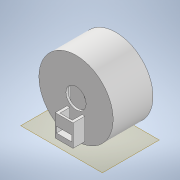
# Autodesk Inventor part: Crank
Saved by Autodesk Inventor 2022.2 (Build 262287000, 287)
## iProperties
Created: 2022-08-12
Part Number: Crank
Material: Generic
Document SubType Name: Modeling
Designer: Ilewicz
Density: 1 g/cm^3
Appearance: Default
r_crank: 15,000 mm
h_tool_holder: 4,000 mm
h_screw_plate: 0,800 mm
r_tool: 2,500 mm
Author: Ilewicz
Autodesk Inventor part; units mm, degrees
ref_plane "YZ Plane" through (0, 0, 0) normal (1, 0, 0) x (0, 1, 0)
ref_plane "XZ Plane" through (0, 0, 0) normal (0, 1, 0) x (-1, 0, 0)
ref_plane "XY Plane" through (0, 0, 0) normal (0, 0, 1) x (1, 0, 0)
derived "Motor.ipt"
sketch "Sketch1" plane through (0, 0, 0) normal (0, 0, 1) x (1, 0, 0)
  line L0 (-3.1964, 3.5) -> (-3.1964, -5.5) construction
  arc A0 (-1.1964, 3.4987) -> (-3.1964, 1.5) centre (-3.1964, 3.5) ccw construction
  line L1 (-5.6964, -1) -> (-5.6964, -3) construction
  line L2 (-0.6964, -3) -> (-0.6964, -1) construction
  arc A1 (-0.6964, -1) -> (-5.6964, -1) centre (-3.1964, -1) ccw construction
  circle A2 centre (-3.1964, 3.5) radius 1.1
  line L3 (2.1036, -3) -> (2.1036, 0)
  arc A3 (4.3036, 0) -> (2.1036, 0) centre (3.2036, 0) ccw
  line L4 (4.3036, 0) -> (4.3036, -3)
  arc A4 (2.1036, -3) -> (4.3036, -3) centre (3.2036, -3) ccw
  line L5 (0.1508, 2.1505) -> (5.7036, 2.1505)
  arc A5 (-1.1964, 3.4987) -> (0.1508, 2.1505) centre (0.1508, 3.4977) ccw
  arc A6 (-1.1964, 3.4987) -> (-3.1964, 1.5) centre (-3.1964, 3.5) ccw
  arc A7 (0.7036, -0.5) -> (-1.2964, 1.5) centre (-1.2964, -0.5) ccw
  line L6 (0.7036, -0.5) -> (0.7036, -3)
  arc A8 (0.7036, -3) -> (5.7036, -3) centre (3.2036, -3) ccw
  line L7 (5.7036, -3) -> (5.7036, 2.1505)
  circle A9 centre (-3.1964, 3.5) radius 1.6 construction
  spline S0 degree 3 poles (-0.0964, 1.1) (-0.2709, 1.2308) (-0.4689, 1.3337) (-0.8824, 1.4687) (-1.0974, 1.5) (-1.2964, 1.5) knots 0 0 0 0 0.5 0.5 1 1 1 1
  line L8 (-3.1964, 1.5) -> (-1.2964, 1.5)
  line L9 (0.4036, -1) -> (0.4036, -11.0616)
  line L10 (-6.7964, -11.0616) -> (-6.7964, -1)
  line L11 (-6.7964, -1) -> (0.4036, -1)
  arc A10 (-6.7964, -11.0616) -> (0.4036, -11.0616) centre (-3.1964, 3.5) ccw
  line L12 (-3.1964, -12.8219) -> (-3.1964, 17.006)
  line L13 (-0.6964, -3) -> (-5.6964, -3) construction
  line L14 (-5.6964, -3) -> (-0.6964, -3) construction
  line L15 (-0.6964, -3) -> (-0.6964, -5.5) construction
  line L16 (-0.6964, -5.5) -> (-5.6964, -5.5) construction
  line L17 (-5.6964, -5.5) -> (-5.6964, -3) construction
  line L18 (-6.2964, -7.9) -> (-0.0964, -7.9)
  line L19 (-0.0964, -7.9) -> (-0.0964, -5.5)
  line L20 (-0.0964, -5.5) -> (-6.2964, -5.5)
  line L21 (-6.2964, -5.5) -> (-6.2964, -7.9)
  line L22 (-6.7964, -9.9) -> (0.4036, -9.9)
  point P0 (0, 0)
  point P1 (-0.6746, 1.4009)
  point P2 (-0.6752, 1.4011)
  point P3 (-3.1964, -11.5)
  point P4 (-3.1964, -11.5)
  dimension "d6" = 3.2
  dimension "r_crank" = 15
  dimension "d51" = 0.3
  dimension "r_tool" = 2.5
  dimension "d53" = 2
  dimension "d55" = 2.5
  dimension "d57" = 6.2
  dimension "d58" = 2.4
  dimension "d90" = 2
  dimension "d91" = 13.4
  constraints: 34 end point, 7 parallel, 6 point on circle, 5 point on line, 4 horizontal, 4 perpendicular, 3 centre point, 3 collinear, 3 tangent, 3 vertical, 2 coincident, 2 midpoint, 3 other
  measures "d6" diameter of A9
  measures "r_crank" radius of A10
  measures "d51" distance between parallel lines of L9 L6
  measures "r_tool" radius of A1
  measures "d53" distance of L1.start L1.end
  measures "d55" distance of L17.end L16.end
  measures "d57" distance of L18.start L18.end
  measures "d58" distance of L20.end L18.start
  measures "d90" distance between parallel lines of L22 L18
  measures "d91" distance from line of L22 A9.centre
extrude "Extrusion1" add sketch "Sketch1" along normal blind 0.8 contours L9 L22 L12 L18 L19 L20 L11 | L12 L20 L21 L18 L22 L10 L11
sketch "Sketch2" plane through (0, 0, 0) normal (0, 0, -1) x (-1, 0, 0)
  line L0 (-0.4036, -9.9) -> (-0.4036, -1) projected
  line L1 (6.7964, -1) -> (6.7964, -9.9) projected
  line L2 (-0.4036, -1) -> (6.7964, -1) projected
  line L3 (0.0964, -5.5) -> (0.0964, -7.9) projected
  line L4 (6.2964, -5.5) -> (0.0964, -5.5) projected
  line L5 (6.2964, -7.9) -> (6.2964, -5.5) projected
  line L6 (0.6964, -3) -> (0.6964, -5.5) projected
  line L7 (0.6964, -3) -> (0.6964, -1) projected
  line L8 (5.6964, -5.5) -> (5.6964, -3) projected
  line L9 (5.6964, -1) -> (5.6964, -3) projected
  line L10 (0.0964, -7.9) -> (6.2964, -7.9) projected
  line L11 (6.7964, -9.9) -> (-0.4036, -9.9) projected
extrude "Extrusion2" add sketch "Sketch2" along normal blind 4 contours L0 L2 L7 L6 L4 L3 L10 L5 L8 L9 L1 L11
sketch "Sketch11" plane through (0, 0, -4) normal (0, 0, -1) x (-1, 0, 0)
  arc A0 (-0.4036, -11.0616) -> (6.7964, -11.0616) centre (3.1964, 3.5) ccw projected
  circle A1 centre (3.1964, 3.5) radius 15
  circle A2 centre (3.1964, 3.5) radius 4.08
  point P0 (0, 0)
  point P1 (6.7964, -11.0616)
  point P2 (-0.4036, -11.0616)
  dimension "d64" = 8.16
  constraints: 2 centre point, 2 coincident
  measures "d64" diameter of A2
extrude "Extrusion8" add sketch "Sketch11" along normal blind 1
sketch "Sketch12" plane through (-3.1964, 3.5, -5) normal (0, 0, -1) x (-1, 0, 0)
  arc A0 (8.16, 0) -> (-8.16, 0) centre (0, 0) ccw
  line L0 (8.16, 0) -> (8.16, -12.5863)
  circle A1 centre (0, 0) radius 15 projected
  line L1 (-8.16, 0) -> (-8.16, -12.5863)
  line L2 (0, -16.3219) -> (0, 13.506) projected
  point P0 (-3.1964, -3.5)
  dimension "d61" = 8.16
  constraints: 4 end point, 4 point on circle, 2 tangent, 1 centre point, 1 coincident, 1 parallel, 1 vertical, 1 other
  measures "d61" radius of A0
extrude "Extrusion9" add sketch "Sketch12" along normal blind 5.1 contours A0 L1 A1 L0
sketch "Sketch13" plane through (-3.1964, 3.5, -10.1) normal (0, 0, -1) x (-1, 0, 0)
  circle A0 centre (0, 0) radius 15
  arc A1 (-8.16, -12.5863) -> (8.16, -12.5863) centre (0, 0) ccw projected
  arc A2 (1.53, -2.04) -> (-1.53, -2.04) centre (0, 0) ccw
  line L0 (1.53, -2.04) -> (-1.53, -2.04)
  line L1 (2.9, -2.04) -> (-2.9, -2.04)
  line L2 (-2.9, -2.04) -> (-2.9, -4.64)
  line L3 (-2.9, -4.64) -> (2.9, -4.64)
  line L4 (2.9, -4.64) -> (2.9, -2.04)
  line L5 (0, -16.3219) -> (0, 13.506) projected
  point P0 (-3.1964, -3.5)
  point P1 (-1.53, -2.04)
  point P2 (1.53, -2.04)
  dimension "d67" = 5.1
  dimension "d68" = 2.04
  dimension "d69" = 5.8
  dimension "d70" = 2.6
  constraints: 10 end point, 2 centre point, 2 coincident, 2 horizontal, 2 parallel, 2 point on circle, 1 collinear, 1 concentric, 1 perpendicular, 1 other
  measures "d67" diameter of A2
  measures "d68" distance from line of L0 A0.centre
  measures "d69" distance of L3.end L2.end
  measures "d70" distance of L2.end L1.end
extrude "Extrusion10" add sketch "Sketch13" along normal blind 10
ref_plane "Work Plane6" through (-3.1964, -11.5, -4) normal (0, -1, 0) x (1, 0, 0)
sketch "Sketch14" plane through (-3.1964, -11.5, -4) normal (0, -1, 0) x (1, 0, 0)
  line L0 (-2.9, -6.1) -> (2.9, -6.1) projected
  line L1 (2.9, -6.1) -> (2.9, -16.1) projected
  line L2 (-2.9, -16.1) -> (2.9, -16.1) projected
  line L3 (-2.9, -6.1) -> (-2.9, -16.1) projected
  line L4 (0, -6.1) -> (2.9, -7.7743)
  line L5 (2.9, -7.7743) -> (2.9, -11.1229)
  line L6 (2.9, -11.1229) -> (0, -12.7973)
  line L7 (0, -12.7973) -> (-2.9, -11.1229)
  line L8 (-2.9, -11.1229) -> (-2.9, -7.7743)
  line L9 (-2.9, -7.7743) -> (0, -6.1)
  point P0 (3.1964, 4)
  point P1 (0, -9.4486)
  constraints: 12 end point, 1 collinear, 1 midpoint, 13 other
hole "Hole2" at (-3.1964, -11.5, -13.4486) direction (0, 1, 0) diameter 3.2 depth 10.36 counterbore diameter 6 counterbore depth 3
sketch "Sketch15" plane through (-3.1964, -11.5, -4) normal (0, -1, 0) x (1, 0, 0)
  line L0 (-3.1, 0) -> (3.1, 0) projected
  line L1 (-3.1, 4) -> (3.1, 4) projected
  line L2 (-2.5, 4) -> (-2.5, 0) construction
  line L3 (0, 4) -> (0, 0) construction
  point P0 (3.1964, 4)
  point P1 (0, 2)
  constraints: 3 midpoint, 2 end point
hole "Hole3" at (-3.1964, -11.5, -2) direction (0, 1, 0) diameter 3.2 depth 3.6
sketch "Sketch16" plane through (-3.1964, 3.5, -10.1) normal (0, 0, 1) x (1, 0, 0)
  arc A0 (1.53, -2.04) -> (-1.53, -2.04) centre (0, 0) ccw projected
  circle A1 centre (0, 0) radius 4.5
  point P0 (3.1964, -3.5)
  dimension "d85" = 9
  constraints: 1 centre point, 1 coincident
  measures "d85" diameter of A1
extrude "Extrusion11" cut sketch "Sketch16" along normal blind 5.25 and the other way blind 0.25
sketch "Sketch17" plane through (-3.1964, 3.5, -4) normal (0, 0, 1) x (1, 0, 0)
  line L0 (-3.6, -4.5) -> (-3.6, -13.4) projected
  line L1 (-3.6, -13.4) -> (3.6, -13.4) projected
  line L2 (3.6, -13.4) -> (3.6, -4.5) projected
  line L3 (3.6, -4.5) -> (-3.6, -4.5) projected
  line L4 (-3.1, -9) -> (3.1, -9) projected
  line L5 (3.1, -9) -> (3.1, -11.4) projected
  line L6 (3.1, -11.4) -> (-3.1, -11.4) projected
  line L7 (-3.1, -11.4) -> (-3.1, -9) projected
  point P0 (3.1964, -3.5)
extrude "Extrusion12" cut sketch "Sketch17" against normal blind 0.6 contours L4 L5 L6 L7
body "Solid1"
